nixal_spoolHolder38 (Autodesk Fusion 360 design; units mm, degrees)
Autodesk Fusion 360 part; units mm, degrees
sketch "Sketch1" plane through (0, 0, 0) normal (0, 1, 0) x (1, 0, 0)
  circle A0 centre (0, 0) radius 11
  circle A1 centre (0, 0) radius 17
  circle A2 centre (0, 0) radius 19
  circle A3 centre (0, 0) radius 30
  dimension "d1" = 22
  dimension "d2" = 34
  dimension "d3" = 38
  dimension "d4" = 60
  constraint coincident A0.centre A1.centre
  constraint concentric A0 A1
  constraint concentric A1 A2
  constraint concentric A2 A3
  measures "d1" diameter of A0
  measures "d2" diameter of A1
  measures "d3" diameter of A2
  measures "d4" diameter of A3
extrude "Extrude4" add sketch "Sketch1" along normal blind 20 contours A1 | A2 | A3
extrude "Extrude5" cut sketch "Sketch1" along normal blind 34 and the other way blind -7 contours A1
extrude "Extrude6" cut sketch "Sketch1" along normal blind 35 and the other way blind -3 contours A3
